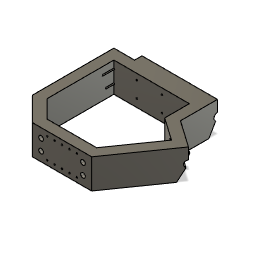
palm (Autodesk Fusion 360 design; units mm, degrees)
Autodesk Fusion 360 part; units mm, degrees
sketch "Sketch1" plane through (0, 0, 0) normal (0, 1, 0) x (1, 0, 0)
  line L0 (0, 0) -> (14, 0)
  line L1 (14, 0) -> (14, 5)
  line L2 (14, 5) -> (65, 5)
  line L3 (65, 5) -> (65, -20)
  line L4 (65, -20) -> (83.0213, -32.6187)
  line L5 (0, 0) -> (0, -55)
  line L6 (0, -55) -> (16.0861, -71.0861)
  line L7 (16.0861, -71.0861) -> (56.0861, -71.0861)
  line L8 (56.0861, -71.0861) -> (83.0213, -32.6187)
  line L9 (7, -7) -> (7, -52.1005)
  line L10 (7, -52.1005) -> (18.9856, -64.0861)
  line L11 (18.9856, -64.0861) -> (52.4422, -64.0861)
  line L12 (52.4422, -64.0861) -> (73.2722, -34.3377)
  line L13 (73.2722, -34.3377) -> (58, -23.644)
  line L14 (58, -23.644) -> (58, -7)
  line L15 (58, -7) -> (7, -7)
  dimension "d15" = 14
  dimension "d16" = 5
  dimension "d17" = 51
  dimension "d18" = 25
  dimension "d19" = 125
  dimension "d22" = 135
  dimension "d23" = 40
  dimension "d25" = 55
  dimension "d27" = 7
  dimension "d28" = 7
  dimension "d29" = 7
  dimension "d30" = 7
  dimension "d31" = 7
  dimension "d32" = 7
  dimension "d33" = 7
  dimension "d34" = 22
  constraint coincident L0.start L5.start
  constraint horizontal L0
  constraint perpendicular L0 L1
  constraint perpendicular L1 L2
  constraint perpendicular L2 L3
  constraint perpendicular L0 L5
  constraint perpendicular L5 L7
  constraint perpendicular L4 L8
  constraint parallel L5 L9
  constraint parallel L6 L10
  constraint parallel L7 L11
  constraint parallel L8 L12
  constraint parallel L4 L13
  constraint parallel L3 L14
  constraint parallel L2 L15
  measures "d15" distance of L0.start L0.end
  measures "d16" distance of L0.end L1.end
  measures "d17" distance of L1.end L2.end
  measures "d18" distance of L2.end L3.end
  measures "d19" angle of L3 L4 L9.end
  measures "d22" angle of L5 L6
  measures "d23" distance of L6.end L7.end
  measures "d25" distance of L0.start L5.end
  measures "d27" distance of L7 L11
  measures "d28" distance of L8 L12
  measures "d29" distance of L4 L13
  measures "d30" distance of L3 L14
  measures "d31" distance of L0 L15
  measures "d32" distance of L5 L9
  measures "d33" distance of L6 L10
  measures "d34" distance of L3.end L4.end L9.end
extrude "Extrude1" add sketch "Sketch1" along normal blind 20
sketch "Sketch2" plane through (0, 0, 0) normal (-1, 0, 0) x (0, 0, 1)
  line L0 (0, 0) -> (55, 0)
  line L1 (55, 0) -> (55, 20)
  line L2 (55, 20) -> (0, 20)
  line L3 (0, 20) -> (0, 0)
  line L4 (0, 10) -> (5.7735, 0)
  line L5 (0, 10) -> (11.547, 10) construction
  circle A0 centre (0, 10) radius 1.2
  circle A1 centre (0, 10) radius 2.2
  circle A2 centre (0, 10) radius 2.4
  dimension "d37" = 60
  dimension "d38" = 2.4
  dimension "d39" = 1
  dimension "d40" = 0.2
  constraint horizontal L5
  constraint midpoint L3 L4.start
  constraint coincident L0 L4.end
  constraint coincident L4.start L5.start
  constraint concentric A0 A1
  constraint concentric A0 A2
  measures "d37" angle of L4 L5
  measures "d38" diameter of A0
  measures "d39" distance of A0 A1
  measures "d40" distance of A1 A2
extrude "Extrude2" cut sketch "Sketch2" against normal up to surface (14 mm away) contours L0 L3 L4 A2 | L3 L4 A1 A2 | L3 L4 A1 A2 | L3 L4 A0 A1 | L3 L4 A0 A1 | L3 L4 A0 | L3 L4 A0
ref_plane "WorkPlane1" through (7, 10, 0.3868) normal (-1, 0, 0) x (0, 0, 1)
extrude "Extrude3" add sketch "Sketch2" along normal mid plane 4 from surface at -7 contours L3 L4 A1 A2 | L3 A0 A1 | L3 L4 A0 A1 | L3 L4 A0 A1 picked at (1.356, 8.1084)
sketch "Sketch3" plane through (71.0339, 0, 49.7385) normal (0.819152, 0, 0.573576) x (0.573576, 0, -0.819152)
  line L0 (-26.0607, 0) -> (20.8994, 0)
  line L1 (20.8994, 0) -> (20.8994, 20)
  line L2 (20.8994, 20) -> (-26.0607, 20)
  line L3 (-26.0607, 20) -> (-26.0607, 0)
  line L4 (20.8994, 10) -> (15.1259, 0)
  line L5 (20.8994, 10) -> (32.4464, 10) construction
  circle A0 centre (20.8994, 10) radius 1.2
  circle A1 centre (20.8994, 10) radius 2.2
  circle A2 centre (20.8994, 10) radius 2.4
  dimension "d46" = 120
  dimension "d47" = 2.4
  dimension "d48" = 1
  dimension "d49" = 0.2
  constraint horizontal L5
  constraint midpoint L1 L4.start
  constraint coincident L0 L4.end
  constraint coincident L4.start L5.start
  constraint concentric A0 A1
  constraint concentric A1 A2
  measures "d46" angle of L4 L5
  measures "d47" diameter of A0
  measures "d48" distance of A0 A1
  measures "d49" distance of A1 A2
extrude "Extrude4" cut sketch "Sketch3" along normal up to surface contours L0 L1 L4 A2 | L1 L4 A1 A2 | L1 L4 A1 A2 | L1 A1 A2 | L1 L4 A0 A1 | L1 L4 A0 A1 | L1 A0 A1 | L1 L4 A0 | L1 L4 A0 | L1 A0 end surface through (65, 0, -5) normal (1, 0, 0) offset 0
ref_plane "WorkPlane2" through (73.6665, 7.8474, 26.8008) normal (0.819152, 0, 0.573576) x (0.573576, 0, -0.819152)
extrude "Extrude5" add sketch "Sketch3" along normal mid plane 4 from surface at -11 contours L1 L4 A1 A2 | L1 L4 A0 A1 | L1 L4 A0 A1 | L1 A0 A1 picked at (20.7835, 12.3249)
sketch "Sketch4" plane through (65, 0, 0) normal (1, 0, 0) x (0, 0, -1)
  line L0 (-27.0481, 0) -> (5, 0)
  line L1 (5, 0) -> (5, 20)
  line L2 (5, 20) -> (-20, 20)
  line L3 (-20, 20) -> (-20, 12.4)
  ellipse E0 centre (-20, 10) end of major axis (-17.0701, 10) minor radius 2.4 (-20, 12.4) -> (-21.4649, 7.9215) ccw
  line L4 (-21.4649, 7.9215) -> (-27.0481, 0)
  line L5 (5, 10) -> (-0.7735, 0)
  line L6 (5, 10) -> (16.547, 10) construction
  circle A0 centre (5, 10) radius 1.2
  circle A1 centre (5, 10) radius 2.2
  circle A2 centre (5, 10) radius 2.4
  dimension "d56" = 120
  dimension "d57" = 2.4
  dimension "d58" = 1
  dimension "d59" = 0.2
  constraint horizontal L6
  constraint midpoint L1 L5.start
  constraint coincident L0 L5.end
  constraint coincident L5.start L6.start
  constraint concentric A0 A1
  constraint concentric A1 A2
  measures "d56" angle of L5 L6
  measures "d57" diameter of A0
  measures "d58" distance of A0 A1
  measures "d59" distance of A1 A2
extrude "Extrude6" cut sketch "Sketch4" against normal up to surface (51 mm away) contours L0 L1 L5 A2 | L1 L5 A1 A2 | L1 L5 A1 A2 | L1 L5 A0 A1 | L1 L5 A0 A1 | L1 L5 A0 | L1 L5 A0
ref_plane "WorkPlane3" through (56.5, 10, 11.0241) normal (1, 0, 0) x (0, 0, -1)
ref_plane "WorkPlane4" through (39.5, 10, 11.0241) normal (1, 0, 0) x (0, 0, -1)
ref_plane "WorkPlane5" through (22.5, 10, 11.0241) normal (1, 0, 0) x (0, 0, -1)
extrude "Extrude7" add sketch "Sketch4" along normal mid plane 4 from surface at -8.5 contours L1 L5 A1 A2 | L1 L5 A0 A1 | L1 L5 A0 A1 | L1 A0 A1 picked at (4.8841, 12.3249)
extrude "Extrude8" add sketch "Sketch4" along normal mid plane 4 from surface at -25.5 contours L1 L5 A1 A2 | L1 L5 A0 A1 | L1 L5 A0 A1 | L1 A0 A1 picked at (4.8841, 12.3249)
extrude "Extrude9" add sketch "Sketch4" along normal mid plane 4 from surface at -42.5 contours L1 L5 A1 A2 | L1 L5 A0 A1 | L1 L5 A0 A1 | L1 A0 A1 picked at (4.8841, 12.3249)
sketch "Sketch5" plane through (60.9629, 10, 44.9436) normal (0.819152, 0, 0.573576) x (0.573576, 0, -0.819152)
  line L0 (0, 7.2746) -> (40.3332, 7.2746) construction
  line L1 (-0.1598, 7.7746) -> (31.4774, 7.7746)
  line L2 (30.8077, -6.3) -> (0, -6.3)
  dimension "d75" = 7.2746
  dimension "d76" = 0.5
  dimension "d77" = 6.3
  constraint horizontal L0
  constraint parallel L0 L1
  constraint horizontal L2
  measures "d75" distance of origin L0
  measures "d76" distance of L0 L1
  measures "d77" distance of origin L2
sketch "Sketch6" plane through (56.5, 10, 11.0241) normal (1, 0, 0) x (0, 0, -1)
  line L0 (0, 5.456) -> (26.4456, 5.456) construction
  line L1 (-0.1606, -4.725) -> (27.0803, -4.725)
  line L2 (-0.1118, 5.956) -> (28.8377, 5.956)
  dimension "d78" = 5.456
  dimension "d79" = 4.725
  dimension "d80" = 0.5
  constraint horizontal L0
  constraint horizontal L1
  constraint horizontal L2
  measures "d78" distance of origin L0
  measures "d79" distance of origin L1
  measures "d80" distance of L0 L2
sketch "Sketch7" plane through (39.5, 10, 11.0241) normal (1, 0, 0) x (0, 0, -1)
  line L0 (0, 5.456) -> (27.2016, 5.456) construction
  line L1 (0, -4.725) -> (27.3227, -4.725)
  line L2 (0, 5.956) -> (27.5044, 5.956)
  dimension "d81" = 5.456
  dimension "d82" = 0.5
  dimension "d83" = 4.725
  constraint horizontal L0
  constraint horizontal L1
  constraint parallel L0 L2
  measures "d81" distance of origin L0
  measures "d82" distance of L0 L2
  measures "d83" distance of origin L1
sketch "Sketch8" plane through (22.5, 10, 11.0241) normal (1, 0, 0) x (0, 0, -1)
  line L0 (0, 5.456) -> (18.9059, 5.456) construction
  line L1 (-0.0823, 5.956) -> (18.8235, 5.956)
  line L2 (0, -4.725) -> (19.1957, -4.725)
  dimension "d84" = 5.456
  dimension "d85" = 0.5
  dimension "d86" = 4.725
  constraint horizontal L0
  constraint parallel L0 L1
  constraint horizontal L2
  measures "d84" distance of origin L0
  measures "d85" distance of L0 L1
  measures "d86" distance of origin L2
sketch "Sketch9" plane through (7, 10, 0.3868) normal (-1, 0, 0) x (0, 0, -1)
  line L0 (3.5821, -4.8648) -> (-14.2183, -4.8648)
  line L1 (4.0225, 3.78) -> (-12.0529, 3.78)
  line L2 (3.5821, -4.3648) -> (3.2151, -4.3648) construction
  line L3 (3.2151, -4.3648) -> (-15.2826, -4.3648) construction
  dimension "d87" = 4.3648
  dimension "d88" = 0.5
  dimension "d89" = 3.78
  constraint horizontal L0
  constraint horizontal L1
  constraint horizontal L2
  constraint parallel L2 L3
  measures "d87" distance of origin L3
  measures "d88" distance of L0 L3
  measures "d89" distance of origin L1
pipe "Pipe1" cut diameter 1 path "Sketch5" along L1
pipe "Pipe2" cut diameter 1 path "Sketch5" along L2
pipe "Pipe3" cut diameter 1 path "Sketch6" along L2
pipe "Pipe4" cut diameter 1 path "Sketch6" along L1
pipe "Pipe5" cut diameter 1 path "Sketch7" along L2
pipe "Pipe6" cut diameter 1 path "Sketch7" along L1
pipe "Pipe7" cut diameter 1 path "Sketch8" along L1
pipe "Pipe8" cut diameter 1 path "Sketch8" along L2
pipe "Pipe9" cut diameter 1 path "Sketch9" along L0
pipe "Pipe10" cut diameter 1 path "Sketch9" along L1
sketch "Sketch10" plane through (0, 0, 71.0861) normal (0, 0, 1) x (1, 0, 0)
  line L0 (16.0861, 0) -> (56.0861, 0)
  line L1 (56.0861, 0) -> (56.0861, 20)
  line L2 (56.0861, 20) -> (16.0861, 20)
  line L3 (16.0861, 20) -> (16.0861, 0)
  line L4 (36.0861, 20) -> (36.0861, 0) construction
  line L5 (36.0861, 17) -> (41.0861, 17) construction
  circle A0 centre (36.0861, 17) radius 0.5
  line L6 (41.0861, 17) -> (46.0861, 17) construction
  line L7 (36.0861, 17) -> (31.0861, 17) construction
  line L8 (31.0861, 17) -> (26.0861, 17) construction
  circle A1 centre (41.0861, 17) radius 0.5
  circle A2 centre (46.0861, 17) radius 0.5
  circle A3 centre (31.0861, 17) radius 0.5
  circle A4 centre (26.0861, 17) radius 0.5
  line L9 (36.0861, 10) -> (56.0861, 10) construction
  circle A5 centre (26.0861, 3) radius 0.5
  circle A6 centre (31.0861, 3) radius 0.5
  circle A7 centre (36.0861, 3) radius 0.5
  circle A8 centre (41.0861, 3) radius 0.5
  circle A9 centre (46.0861, 3) radius 0.5
  dimension "d130" = 5
  dimension "d132" = 1
  dimension "d133" = 3
  dimension "d134" = 1
  dimension "d135" = 1
  dimension "d136" = 1
  dimension "d137" = 1
  constraint midpoint L2 L4.start
  constraint midpoint L0 L4.end
  constraint coincident L4 L5.start
  constraint perpendicular L4 L5
  constraint coincident L5.start A0.centre
  constraint perpendicular L1 L6
  constraint equal L5 L6
  constraint perpendicular L4 L7
  constraint perpendicular L4 L8
  constraint equal L5 L7
  constraint equal L7 L8
  constraint coincident L5.end L6.start
  constraint coincident L6.end A2.centre
  constraint coincident L7.end L8.start
  constraint coincident L8.end A4.centre
  constraint midpoint L4 L9.start
  constraint midpoint L1 L9.end
  constraint symmetric A0 L9 A7
  constraint symmetric A1 L9 A8
  constraint symmetric A2 L9 A9
  constraint symmetric A3 L9 A6
  constraint symmetric A4 L9 A5
  measures "d130" distance of L5.start L5.end
  measures "d132" diameter of A0
  measures "d133" distance of L2 L5.start
  measures "d134" diameter of A1
  measures "d135" diameter of A2
  measures "d136" diameter of A3
  measures "d137" diameter of A4
extrude "Extrude10" cut sketch "Sketch10" against normal up to surface (7 mm away) contours A0 | A1 | A2 | A3 | A4 | A5 | A6 | A7 | A8 | A9
sketch "Sketch11" plane through (0, 0, 71.0861) normal (0, 0, 1) x (1, 0, 0)
  circle A0 centre (36.0861, 17) radius 0.5
  circle A1 centre (41.0861, 3) radius 0.5
  circle A2 centre (26.0861, 3) radius 0.5
  circle A3 centre (46.0861, 3) radius 0.5
  circle A4 centre (31.0861, 17) radius 0.5
  circle A5 centre (41.0861, 17) radius 0.5
  circle A6 centre (36.0861, 3) radius 0.5
  circle A7 centre (31.0861, 3) radius 0.5
  circle A8 centre (46.0861, 17) radius 0.5
  circle A9 centre (26.0861, 17) radius 0.5
  line L0 (16.0861, 0) -> (56.0861, 0)
  line L1 (56.0861, 0) -> (56.0861, 20)
  line L2 (56.0861, 20) -> (16.0861, 20)
  line L3 (16.0861, 20) -> (16.0861, 0)
  line L4 (26.0861, 17) -> (26.0861, 3) construction
  line L5 (26.0861, 10) -> (21.9361, 10) construction
  line L6 (21.9361, 10) -> (21.9361, 13.75) construction
  circle A10 centre (21.9361, 13.75) radius 1.6
  line L7 (36.0861, 17) -> (36.0861, 3) construction
  line L8 (24.4361, 15.1934) -> (21.9361, 16.6368)
  line L9 (21.9361, 16.6368) -> (19.4361, 15.1934)
  line L10 (19.4361, 15.1934) -> (19.4361, 12.3066)
  line L11 (19.4361, 12.3066) -> (21.9361, 10.8632)
  line L12 (21.9361, 10.8632) -> (24.4361, 12.3066)
  line L13 (24.4361, 12.3066) -> (24.4361, 15.1934)
  circle A11 centre (21.9361, 6.25) radius 1.6
  line L14 (24.4361, 4.8066) -> (21.9361, 3.3632)
  line L15 (24.4361, 7.6934) -> (24.4361, 4.8066)
  line L16 (21.9361, 9.1368) -> (24.4361, 7.6934)
  line L17 (19.4361, 7.6934) -> (21.9361, 9.1368)
  line L18 (19.4361, 4.8066) -> (19.4361, 7.6934)
  line L19 (21.9361, 3.3632) -> (19.4361, 4.8066)
  circle A12 centre (50.2361, 6.25) radius 1.6
  line L20 (50.2361, 9.1368) -> (47.7361, 7.6934)
  line L21 (52.7361, 7.6934) -> (50.2361, 9.1368)
  line L22 (52.7361, 4.8066) -> (52.7361, 7.6934)
  line L23 (50.2361, 3.3632) -> (52.7361, 4.8066)
  line L24 (47.7361, 4.8066) -> (50.2361, 3.3632)
  line L25 (47.7361, 7.6934) -> (47.7361, 4.8066)
  line L26 (50.2361, 10.8632) -> (47.7361, 12.3066)
  line L27 (47.7361, 12.3066) -> (47.7361, 15.1934)
  line L28 (47.7361, 15.1934) -> (50.2361, 16.6368)
  line L29 (50.2361, 16.6368) -> (52.7361, 15.1934)
  line L30 (52.7361, 15.1934) -> (52.7361, 12.3066)
  line L31 (52.7361, 12.3066) -> (50.2361, 10.8632)
  circle A13 centre (50.2361, 13.75) radius 1.6
  point P0 (21.9361, 13.75)
  dimension "d141" = 4.15
  dimension "d142" = 3.75
  dimension "d143" = 3.2
  dimension "d144" = 2.5
  constraint coincident A9.centre L4.start
  constraint coincident A2.centre L4.end
  constraint midpoint L4 L5.start
  constraint perpendicular L4 L5
  constraint perpendicular L5 L6
  constraint coincident P0 L6.end
  constraint coincident A0.centre L7.start
  constraint coincident A6.centre L7.end
  constraint symmetric L5 A10 A11
  constraint symmetric L5 L8.start L14.start
  constraint symmetric L5 L8.end L14.end
  constraint symmetric L5 L9.end L18.start
  constraint symmetric L5 L10.end L17.start
  constraint symmetric L5 L11.end L16.start
  constraint symmetric L5 L12.end L15.start
  constraint symmetric A10 L7 A13
  constraint symmetric L7 L8.start L27.end
  constraint symmetric L7 L8.end L28.end
  constraint symmetric L7 L9.end L29.end
  constraint symmetric L7 L10.end L30.end
  constraint symmetric L7 L11.end L26.start
  constraint symmetric L7 L12.end L26.end
  constraint symmetric L7 A11 A12
  constraint symmetric L7 L14.start L24.start
  constraint symmetric L7 L14.end L23.start
  constraint symmetric L7 L15.start L20.end
  constraint symmetric L7 L16.start L20.start
  constraint symmetric L7 L17.start L21.start
  constraint symmetric L7 L18.start L22.start
  measures "d141" distance of L5.start L5.end
  measures "d142" distance of L5.end P0
  measures "d143" diameter of A10
  measures "d144" distance of P0 L13
extrude "Extrude11" cut sketch "Sketch11" against normal blind 21 contours A10 | A11 | A12 | A13
extrude "Extrude12" cut sketch "Sketch11" against normal blind 14 from surface at -3 contours L8 L9 L10 L11 L12 L13 | L14 L15 L16 L17 L18 L19 | L20 L21 L22 L23 L24 L25 | L26 L27 L28 L29 L30 L31
equation "pinkyWidth = 12 mm"
equation "normalWidth = 15 mm"
equation "thumbWidth = 20 mm"
equation "bendingAngle = 30 deg"
equation "toothpickWidth = 2.4 mm"
equation "stringWidth = 1 mm"
equation "clearance = 0.2 mm"
equation "int_eccentricity = 0.63"
equation "ext_eccentricity = int_eccentricity / cos(bendingAngle)"
equation "thumbVSpace = 25 mm"
equation "pinkyVSpace = 5 mm"
equation "wristWidth = 40 mm"
equation "fingerHSpace = 1 mm"
equation "d15 = pinkyWidth + 1 mm + fingerHSpace"
equation "d16 = pinkyVSpace"
equation "d17 = ( normalWidth + 1 mm + fingerHSpace ) * 3"
equation "d18 = thumbVSpace"
equation "d19 = 90 deg + thumbAngle"
equation "thumbAngle = 35 deg"
equation "d22 = 90 deg + 45 deg"
equation "d23 = wristWidth"
equation "leftLength = 55 mm"
equation "d25 = leftLength"
equation "bordersThickness = 7 mm"
equation "d27 = bordersThickness"
equation "d28 = bordersThickness"
equation "d29 = bordersThickness"
equation "d30 = bordersThickness"
equation "d31 = bordersThickness"
equation "d32 = bordersThickness"
equation "d33 = bordersThickness"
equation "d34 = thumbWidth + 1 mm + fingerHSpace"
equation "d35 = thumbWidth"
equation "d37 = 90 deg - bendingAngle"
equation "d38 = toothpickWidth"
equation "d40 = clearance"
equation "d46 = 90 deg + bendingAngle"
equation "d47 = toothpickWidth"
equation "d49 = clearance"
equation "d52 = -( thumbWidth + 1 mm + fingerHSpace ) / 2"
equation "d56 = 90 deg + bendingAngle"
equation "d57 = toothpickWidth"
equation "d59 = clearance"
equation "d62 = -( normalWidth + 1 mm + fingerHSpace ) / 2"
equation "d63 = -( normalWidth + 1 mm + fingerHSpace )"
equation "d64 = -( normalWidth + 1 mm + fingerHSpace )"
equation "d75 = ext_eccentricity * thumbWidth / 2"
equation "d76 = stringWidth / 2"
equation "d77 = int_eccentricity * thumbWidth / 2"
equation "d78 = ext_eccentricity * normalWidth / 2"
equation "d79 = int_eccentricity * normalWidth / 2"
equation "d80 = stringWidth / 2"
equation "d81 = ext_eccentricity * normalWidth / 2"
equation "d82 = stringWidth / 2"
equation "d83 = int_eccentricity * normalWidth / 2"
equation "d84 = ext_eccentricity * normalWidth / 2"
equation "d85 = stringWidth / 2"
equation "d86 = int_eccentricity * normalWidth / 2"
equation "d87 = ext_eccentricity * pinkyWidth / 2"
equation "d88 = stringWidth / 2"
equation "d89 = int_eccentricity * pinkyWidth / 2"
equation "d92 = stringWidth"
equation "d96 = stringWidth"
equation "d100 = stringWidth"
equation "d104 = stringWidth"
equation "d108 = stringWidth"
equation "d112 = stringWidth"
equation "d116 = stringWidth"
equation "d120 = stringWidth"
equation "d124 = stringWidth"
equation "d128 = stringWidth"
equation "d130 = motorSpacing"
equation "motorSpacing = 5 mm"
equation "d132 = stringWidth"
equation "d134 = stringWidth"
equation "d135 = stringWidth"
equation "d136 = stringWidth"
equation "d137 = stringWidth"
named bodies: "palm"
